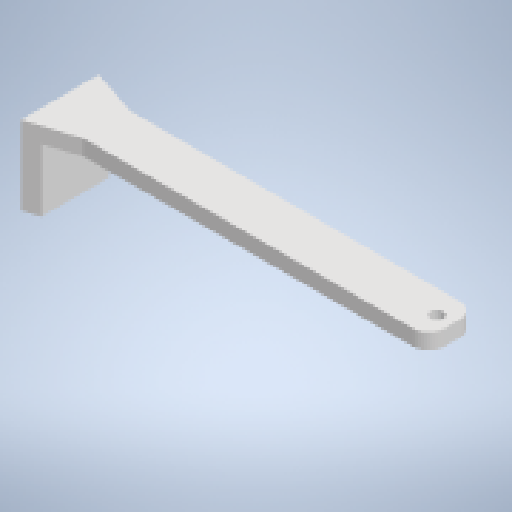
# Autodesk Inventor part: porta penna
Saved by Autodesk Inventor 2024 (Build 280153000, 153)
## iProperties
Created: 2023-12-23
Part Number: porta penna
Material: Generico
Document SubType Name: Modeling
Designer: Giorgio
Density: 1 g/cm^3
Appearance: Default
Author: Giorgio
Autodesk Inventor part; units mm, degrees
ref_plane "YZ Plane" through (0, 0, 0) normal (1, 0, 0) x (0, 1, 0)
ref_plane "XZ Plane" through (0, 0, 0) normal (0, 1, 0) x (-1, 0, 0)
ref_plane "XY Plane" through (0, 0, 0) normal (0, 0, 1) x (1, 0, 0)
sketch "Schizzo1" plane through (0, 0, 0) normal (0, 0, 1) x (1, 0, 0)
  line L0 (0, 0) -> (0, 50)
  line L1 (0, 50) -> (250, 50)
  line L2 (250, 50) -> (250, 40)
  line L3 (250, 40) -> (10, 40)
  line L4 (10, 40) -> (10, 0)
  line L5 (10, 0) -> (0, 0)
  dimension "d0" = 10
  dimension "d1" = 10
  dimension "d2" = 50
  dimension "d3" = 250
  constraints: 12 end point, 4 perpendicular, 1 horizontal, 1 vertical
  measures "d0" distance of L4.end L0.start
  measures "d1" distance of L1.end L2.end
  measures "d2" distance of L0.start L0.end
  measures "d3" distance of L0.end L1.end
extrude "Estrusione1" add sketch "Schizzo1" along normal blind 30
sketch "Schizzo2" plane through (0, 50, 0) normal (0, 1, 0) x (1, 0, 0)
  circle A0 centre (240, -15) radius 4
  line L0 (250, -30) -> (0, -30) projected
  line L1 (250, 0) -> (250, -30) projected
  line L2 (30, 51) -> (328, 51)
  line L3 (328, 51) -> (328, -5)
  line L4 (328, -5) -> (30, -5)
  line L5 (30, 0) -> (30, 51)
  line L6 (336, -124) -> (30, -124)
  line L7 (30, -124) -> (30, -30)
  line L8 (30, -25) -> (336, -25)
  line L9 (336, -25) -> (336, -124)
  line L10 (250, 0) -> (0, 0) projected
  line L11 (0, 0) -> (0, -30) projected
  line L12 (30, -5) -> (0, 0)
  line L13 (30, -25) -> (0, -30)
  line L14 (0, 0) -> (328, 124)
  line L15 (328, 124) -> (336, -220)
  line L16 (336, -220) -> (0, -30)
  point P0 (250, -5)
  point P1 (250, -25)
  dimension "d6" = 8
  dimension "d7" = 15
  dimension "d8" = 10
  dimension "d9" = 5
  dimension "d10" = 5
  dimension "d11" = 30
  constraints: 26 end point, 4 parallel, 3 point on line, 2 horizontal, 2 perpendicular, 1 centre point
  measures "d6" diameter of A0
  measures "d7" distance from line of A0.centre L0
  measures "d8" distance from line of A0.centre L1
  measures "d9" distance between parallel lines of L8 L0
  measures "d10" distance between parallel lines of L10 L4
  measures "d11" distance between parallel lines of L5 L11
extrude "Estrusione2" cut sketch "Schizzo2" against normal blind 50 contours A0 | L0 L13 L8 L1 | L4 L12 L10 L1
fillet "Raccordo1" radius 10 2 edges at (250, 45, 5) (250, 45, 25)
